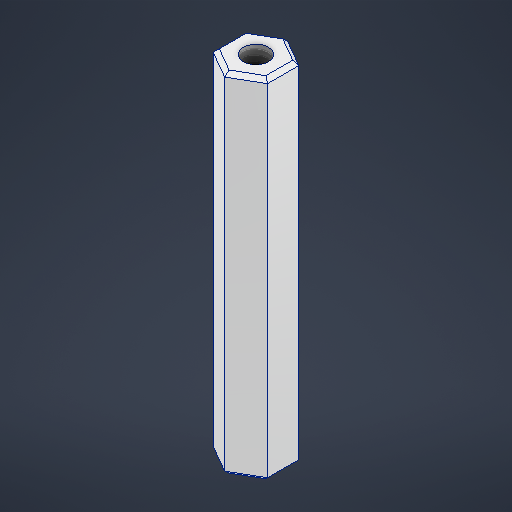
# Autodesk Inventor part: Abstandsbolzen 45mm
Saved by Autodesk Inventor 2025.2 (Build 292293000, 293)
## iProperties
Created: 2024-03-05
Part Number: Abstandsbolzen 45mm
Material: Aluminium 6061
Document SubType Name: Modeling
Designer: Fabian
Density: 2.7 g/cm^3
Appearance: Aluminium - flach
Author: Fabian
Autodesk Inventor part; units mm, degrees
ref_plane "YZ Plane" through (0, 0, 0) normal (1, 0, 0) x (0, 1, 0)
ref_plane "XZ Plane" through (0, 0, 0) normal (0, 1, 0) x (-1, 0, 0)
ref_plane "XY Plane" through (0, 0, 0) normal (0, 0, 1) x (1, 0, 0)
sketch "Skizze1" plane through (0, 0, 0) normal (0, 1, 0) x (-1, 0, 0)
  line L0 (3.5, -2.0207) -> (0, -4.0415)
  line L1 (0, -4.0415) -> (-3.5, -2.0207)
  line L2 (-3.5, -2.0207) -> (-3.5, 2.0207)
  line L3 (-3.5, 2.0207) -> (0, 4.0415)
  line L4 (0, 4.0415) -> (3.5, 2.0207)
  line L5 (3.5, 2.0207) -> (3.5, -2.0207)
  point P0 (0, 0)
  point P1 (0, 0)
  dimension "d0" = 7
  constraints: 12 end point, 1 coincident, 13 other
  measures "d0" distance between parallel lines of L2 L5
extrude "Extrusion1" add sketch "Skizze1" along normal blind 45
sketch "Skizze2" plane through (0, 45, 0) normal (0, 1, 0) x (1, 0, 0)
  point P0 (0, 0)
  point P1 (0, 0)
  constraints: 1 coincident
hole "Bohrung1" at (0, 45, 0) direction (0, -1, 0) diameter 3.242 depth 11.8 tip angle 118 thread size "M4x0.7" class "6H" standard "ISO Metric profile"
sketch "Skizze3" plane through (0, 0, 0) normal (0, -1, 0) x (1, 0, 0)
  point P0 (0, 0)
  point P1 (0, 0)
  constraints: 1 coincident
hole "Bohrung2" at (0, 0, 0) direction (0, 1, 0) diameter 3.242 depth 11.8 tip angle 118 thread size "M4x0.7" class "6H" standard "ISO Metric profile"
chamfer "Fasen1" distance 0.5 angle 45 12 edges at (-1.75, 45, 3.0311) (1.75, 45, 3.0311) (3.5, 45, 0) (1.75, 45, -3.0311) (-1.75, 45, -3.0311) (-3.5, 45, 0) (-3.5, 0, 0) (-1.75, 0, 3.0311) (1.75, 0, 3.0311) (3.5, 0, 0) (1.75, 0, -3.0311) (-1.75, 0, -3.0311)
